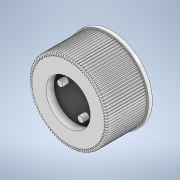
# Autodesk Inventor part: 100ml Bottle 2 lid
Saved by Autodesk Inventor 2021 (Build 250183000, 183)
## iProperties
Created: 2019-11-05
Part Number: 100ml Bottle 2 lid
Material: Generic
Document SubType Name: Modeling
Designer: jgray
Density: 1 g/cm^3
Appearance: Default
Author: jgray
Autodesk Inventor part; units mm, degrees
ref_plane "YZ Plane" through (0, 0, 0) normal (1, 0, 0) x (0, 1, 0)
ref_plane "XZ Plane" through (0, 0, 0) normal (0, 1, 0) x (-1, 0, 0)
ref_plane "XY Plane" through (0, 0, 0) normal (0, 0, 1) x (1, 0, 0)
sketch "Sketch1" plane through (0, 0, 0) normal (0, 0, 1) x (1, 0, 0)
  circle A0 centre (0, 0) radius 13.8
  dimension "d0" = 27.6
  constraints: 1 centre point, 1 coincident
  measures "d0" diameter of A0
extrude "Extrusion1" add sketch "Sketch1" along normal blind 1.3
sketch "Sketch2" plane through (0, 0, 1.3) normal (0, 0, 1) x (1, 0, 0)
  circle A0 centre (0, 0) radius 13.4
  circle A1 centre (0, 0) radius 12.9 construction
  line L0 (0, 13.4) -> (0.8414, 13.3736) construction
  line L1 (0.8414, 13.3736) -> (1.6795, 13.2943) construction
  line L2 (1.6795, 13.2943) -> (2.5109, 13.1626) construction
  line L3 (2.5109, 13.1626) -> (3.3324, 12.979) construction
  line L4 (3.3324, 12.979) -> (4.1408, 12.7442) construction
  line L5 (4.1408, 12.7442) -> (4.9329, 12.459) construction
  line L6 (4.9329, 12.459) -> (5.7054, 12.1247) construction
  line L7 (5.7054, 12.1247) -> (6.4555, 11.7425) construction
  line L8 (6.4555, 11.7425) -> (7.1801, 11.314) construction
  line L9 (7.1801, 11.314) -> (7.8763, 10.8408) construction
  line L10 (7.8763, 10.8408) -> (8.5415, 10.3249) construction
  line L11 (8.5415, 10.3249) -> (9.1729, 9.7682) construction
  line L12 (9.1729, 9.7682) -> (9.7682, 9.1729) construction
  line L13 (9.7682, 9.1729) -> (10.3249, 8.5415) construction
  line L14 (10.3249, 8.5415) -> (10.8408, 7.8763) construction
  line L15 (10.8408, 7.8763) -> (11.314, 7.1801) construction
  line L16 (11.314, 7.1801) -> (11.7425, 6.4555) construction
  line L17 (11.7425, 6.4555) -> (12.1247, 5.7054) construction
  line L18 (12.1247, 5.7054) -> (12.459, 4.9329) construction
  line L19 (12.459, 4.9329) -> (12.7442, 4.1408) construction
  line L20 (12.7442, 4.1408) -> (12.979, 3.3324) construction
  line L21 (12.979, 3.3324) -> (13.1626, 2.5109) construction
  line L22 (13.1626, 2.5109) -> (13.2943, 1.6795) construction
  line L23 (13.2943, 1.6795) -> (13.3736, 0.8414) construction
  line L24 (13.3736, 0.8414) -> (13.4, 0) construction
  line L25 (13.4, 0) -> (13.3736, -0.8414) construction
  line L26 (13.3736, -0.8414) -> (13.2943, -1.6795) construction
  line L27 (13.2943, -1.6795) -> (13.1626, -2.5109) construction
  line L28 (13.1626, -2.5109) -> (12.979, -3.3324) construction
  line L29 (12.979, -3.3324) -> (12.7442, -4.1408) construction
  line L30 (12.7442, -4.1408) -> (12.459, -4.9329) construction
  line L31 (12.459, -4.9329) -> (12.1247, -5.7054) construction
  line L32 (12.1247, -5.7054) -> (11.7425, -6.4555) construction
  line L33 (11.7425, -6.4555) -> (11.314, -7.1801) construction
  line L34 (11.314, -7.1801) -> (10.8408, -7.8763) construction
  line L35 (10.8408, -7.8763) -> (10.3249, -8.5415) construction
  line L36 (10.3249, -8.5415) -> (9.7682, -9.1729) construction
  line L37 (9.7682, -9.1729) -> (9.1729, -9.7682) construction
  line L38 (9.1729, -9.7682) -> (8.5415, -10.3249) construction
  line L39 (8.5415, -10.3249) -> (7.8763, -10.8408) construction
  line L40 (7.8763, -10.8408) -> (7.1801, -11.314) construction
  line L41 (7.1801, -11.314) -> (6.4555, -11.7425) construction
  line L42 (6.4555, -11.7425) -> (5.7054, -12.1247) construction
  line L43 (5.7054, -12.1247) -> (4.9329, -12.459) construction
  line L44 (4.9329, -12.459) -> (4.1408, -12.7442) construction
  line L45 (4.1408, -12.7442) -> (3.3324, -12.979) construction
  line L46 (3.3324, -12.979) -> (2.5109, -13.1626) construction
  line L47 (2.5109, -13.1626) -> (1.6795, -13.2943) construction
  line L48 (1.6795, -13.2943) -> (0.8414, -13.3736) construction
  line L49 (0.8414, -13.3736) -> (0, -13.4) construction
  line L50 (0, -13.4) -> (-0.8414, -13.3736) construction
  line L51 (-0.8414, -13.3736) -> (-1.6795, -13.2943) construction
  line L52 (-1.6795, -13.2943) -> (-2.5109, -13.1626) construction
  line L53 (-2.5109, -13.1626) -> (-3.3324, -12.979) construction
  line L54 (-3.3324, -12.979) -> (-4.1408, -12.7442) construction
  line L55 (-4.1408, -12.7442) -> (-4.9329, -12.459) construction
  line L56 (-4.9329, -12.459) -> (-5.7054, -12.1247) construction
  line L57 (-5.7054, -12.1247) -> (-6.4555, -11.7425) construction
  line L58 (-6.4555, -11.7425) -> (-7.1801, -11.314) construction
  line L59 (-7.1801, -11.314) -> (-7.8763, -10.8408) construction
  line L60 (-7.8763, -10.8408) -> (-8.5415, -10.3249) construction
  line L61 (-8.5415, -10.3249) -> (-9.1729, -9.7682) construction
  line L62 (-9.1729, -9.7682) -> (-9.7682, -9.1729) construction
  line L63 (-9.7682, -9.1729) -> (-10.3249, -8.5415) construction
  line L64 (-10.3249, -8.5415) -> (-10.8408, -7.8763) construction
  line L65 (-10.8408, -7.8763) -> (-11.314, -7.1801) construction
  line L66 (-11.314, -7.1801) -> (-11.7425, -6.4555) construction
  line L67 (-11.7425, -6.4555) -> (-12.1247, -5.7054) construction
  line L68 (-12.1247, -5.7054) -> (-12.459, -4.9329) construction
  line L69 (-12.459, -4.9329) -> (-12.7442, -4.1408) construction
  line L70 (-12.7442, -4.1408) -> (-12.979, -3.3324) construction
  line L71 (-12.979, -3.3324) -> (-13.1626, -2.5109) construction
  line L72 (-13.1626, -2.5109) -> (-13.2943, -1.6795) construction
  line L73 (-13.2943, -1.6795) -> (-13.3736, -0.8414) construction
  line L74 (-13.3736, -0.8414) -> (-13.4, 0) construction
  line L75 (-13.4, 0) -> (-13.3736, 0.8414) construction
  line L76 (-13.3736, 0.8414) -> (-13.2943, 1.6795) construction
  line L77 (-13.2943, 1.6795) -> (-13.1626, 2.5109) construction
  line L78 (-13.1626, 2.5109) -> (-12.979, 3.3324) construction
  line L79 (-12.979, 3.3324) -> (-12.7442, 4.1408) construction
  line L80 (-12.7442, 4.1408) -> (-12.459, 4.9329) construction
  line L81 (-12.459, 4.9329) -> (-12.1247, 5.7054) construction
  line L82 (-12.1247, 5.7054) -> (-11.7425, 6.4555) construction
  line L83 (-11.7425, 6.4555) -> (-11.314, 7.1801) construction
  line L84 (-11.314, 7.1801) -> (-10.8408, 7.8763) construction
  line L85 (-10.8408, 7.8763) -> (-10.3249, 8.5415) construction
  line L86 (-10.3249, 8.5415) -> (-9.7682, 9.1729) construction
  line L87 (-9.7682, 9.1729) -> (-9.1729, 9.7682) construction
  line L88 (-9.1729, 9.7682) -> (-8.5415, 10.3249) construction
  line L89 (-8.5415, 10.3249) -> (-7.8763, 10.8408) construction
  line L90 (-7.8763, 10.8408) -> (-7.1801, 11.314) construction
  line L91 (-7.1801, 11.314) -> (-6.4555, 11.7425) construction
  line L92 (-6.4555, 11.7425) -> (-5.7054, 12.1247) construction
  line L93 (-5.7054, 12.1247) -> (-4.9329, 12.459) construction
  line L94 (-4.9329, 12.459) -> (-4.1408, 12.7442) construction
  line L95 (-4.1408, 12.7442) -> (-3.3324, 12.979) construction
  line L96 (-3.3324, 12.979) -> (-2.5109, 13.1626) construction
  line L97 (-2.5109, 13.1626) -> (-1.6795, 13.2943) construction
  line L98 (-1.6795, 13.2943) -> (-0.8414, 13.3736) construction
  line L99 (-0.8414, 13.3736) -> (0, 13.4) construction
  line L100 (0, 0) -> (-0.4207, 13.3868) construction
  line L101 (-0.4052, 12.8936) -> (0.4052, 12.8936) construction
  line L102 (0.4052, 12.8936) -> (1.214, 12.8427) construction
  line L103 (1.214, 12.8427) -> (2.018, 12.7412) construction
  line L104 (2.018, 12.7412) -> (2.814, 12.5893) construction
  line L105 (2.814, 12.5893) -> (3.599, 12.3878) construction
  line L106 (3.599, 12.3878) -> (4.3697, 12.1374) construction
  line L107 (4.3697, 12.1374) -> (5.1232, 11.839) construction
  line L108 (5.1232, 11.839) -> (5.8565, 11.494) construction
  line L109 (5.8565, 11.494) -> (6.5666, 11.1036) construction
  line L110 (6.5666, 11.1036) -> (7.2509, 10.6693) construction
  line L111 (7.2509, 10.6693) -> (7.9065, 10.193) construction
  line L112 (7.9065, 10.193) -> (8.5309, 9.6764) construction
  line L113 (8.5309, 9.6764) -> (9.1217, 9.1217) construction
  line L114 (9.1217, 9.1217) -> (9.6764, 8.5309) construction
  line L115 (9.6764, 8.5309) -> (10.193, 7.9065) construction
  line L116 (10.193, 7.9065) -> (10.6693, 7.2509) construction
  line L117 (10.6693, 7.2509) -> (11.1036, 6.5666) construction
  line L118 (11.1036, 6.5666) -> (11.494, 5.8565) construction
  line L119 (11.494, 5.8565) -> (11.839, 5.1232) construction
  line L120 (11.839, 5.1232) -> (12.1374, 4.3697) construction
  line L121 (12.1374, 4.3697) -> (12.3878, 3.599) construction
  line L122 (12.3878, 3.599) -> (12.5893, 2.814) construction
  line L123 (12.5893, 2.814) -> (12.7412, 2.018) construction
  line L124 (12.7412, 2.018) -> (12.8427, 1.214) construction
  line L125 (12.8427, 1.214) -> (12.8936, 0.4052) construction
  line L126 (12.8936, 0.4052) -> (12.8936, -0.4052) construction
  line L127 (12.8936, -0.4052) -> (12.8427, -1.214) construction
  line L128 (12.8427, -1.214) -> (12.7412, -2.018) construction
  line L129 (12.7412, -2.018) -> (12.5893, -2.814) construction
  line L130 (12.5893, -2.814) -> (12.3878, -3.599) construction
  line L131 (12.3878, -3.599) -> (12.1374, -4.3697) construction
  line L132 (12.1374, -4.3697) -> (11.839, -5.1232) construction
  line L133 (11.839, -5.1232) -> (11.494, -5.8565) construction
  line L134 (11.494, -5.8565) -> (11.1036, -6.5666) construction
  line L135 (11.1036, -6.5666) -> (10.6693, -7.2509) construction
  line L136 (10.6693, -7.2509) -> (10.193, -7.9065) construction
  line L137 (10.193, -7.9065) -> (9.6764, -8.5309) construction
  line L138 (9.6764, -8.5309) -> (9.1217, -9.1217) construction
  line L139 (9.1217, -9.1217) -> (8.5309, -9.6764) construction
  line L140 (8.5309, -9.6764) -> (7.9065, -10.193) construction
  line L141 (7.9065, -10.193) -> (7.2509, -10.6693) construction
  line L142 (7.2509, -10.6693) -> (6.5666, -11.1036) construction
  line L143 (6.5666, -11.1036) -> (5.8565, -11.494) construction
  line L144 (5.8565, -11.494) -> (5.1232, -11.839) construction
  line L145 (5.1232, -11.839) -> (4.3697, -12.1374) construction
  line L146 (4.3697, -12.1374) -> (3.599, -12.3878) construction
  line L147 (3.599, -12.3878) -> (2.814, -12.5893) construction
  line L148 (2.814, -12.5893) -> (2.018, -12.7412) construction
  line L149 (2.018, -12.7412) -> (1.214, -12.8427) construction
  line L150 (1.214, -12.8427) -> (0.4052, -12.8936) construction
  line L151 (0.4052, -12.8936) -> (-0.4052, -12.8936) construction
  line L152 (-0.4052, -12.8936) -> (-1.214, -12.8427) construction
  line L153 (-1.214, -12.8427) -> (-2.018, -12.7412) construction
  line L154 (-2.018, -12.7412) -> (-2.814, -12.5893) construction
  line L155 (-2.814, -12.5893) -> (-3.599, -12.3878) construction
  line L156 (-3.599, -12.3878) -> (-4.3697, -12.1374) construction
  line L157 (-4.3697, -12.1374) -> (-5.1232, -11.839) construction
  line L158 (-5.1232, -11.839) -> (-5.8565, -11.494) construction
  line L159 (-5.8565, -11.494) -> (-6.5666, -11.1036) construction
  line L160 (-6.5666, -11.1036) -> (-7.2509, -10.6693) construction
  line L161 (-7.2509, -10.6693) -> (-7.9065, -10.193) construction
  line L162 (-7.9065, -10.193) -> (-8.5309, -9.6764) construction
  line L163 (-8.5309, -9.6764) -> (-9.1217, -9.1217) construction
  line L164 (-9.1217, -9.1217) -> (-9.6764, -8.5309) construction
  line L165 (-9.6764, -8.5309) -> (-10.193, -7.9065) construction
  line L166 (-10.193, -7.9065) -> (-10.6693, -7.2509) construction
  line L167 (-10.6693, -7.2509) -> (-11.1036, -6.5666) construction
  line L168 (-11.1036, -6.5666) -> (-11.494, -5.8565) construction
  line L169 (-11.494, -5.8565) -> (-11.839, -5.1232) construction
  line L170 (-11.839, -5.1232) -> (-12.1374, -4.3697) construction
  line L171 (-12.1374, -4.3697) -> (-12.3878, -3.599) construction
  line L172 (-12.3878, -3.599) -> (-12.5893, -2.814) construction
  line L173 (-12.5893, -2.814) -> (-12.7412, -2.018) construction
  line L174 (-12.7412, -2.018) -> (-12.8427, -1.214) construction
  line L175 (-12.8427, -1.214) -> (-12.8936, -0.4052) construction
  line L176 (-12.8936, -0.4052) -> (-12.8936, 0.4052) construction
  line L177 (-12.8936, 0.4052) -> (-12.8427, 1.214) construction
  line L178 (-12.8427, 1.214) -> (-12.7412, 2.018) construction
  line L179 (-12.7412, 2.018) -> (-12.5893, 2.814) construction
  line L180 (-12.5893, 2.814) -> (-12.3878, 3.599) construction
  line L181 (-12.3878, 3.599) -> (-12.1374, 4.3697) construction
  line L182 (-12.1374, 4.3697) -> (-11.839, 5.1232) construction
  line L183 (-11.839, 5.1232) -> (-11.494, 5.8565) construction
  line L184 (-11.494, 5.8565) -> (-11.1036, 6.5666) construction
  line L185 (-11.1036, 6.5666) -> (-10.6693, 7.2509) construction
  line L186 (-10.6693, 7.2509) -> (-10.193, 7.9065) construction
  line L187 (-10.193, 7.9065) -> (-9.6764, 8.5309) construction
  line L188 (-9.6764, 8.5309) -> (-9.1217, 9.1217) construction
  line L189 (-9.1217, 9.1217) -> (-8.5309, 9.6764) construction
  line L190 (-8.5309, 9.6764) -> (-7.9065, 10.193) construction
  line L191 (-7.9065, 10.193) -> (-7.2509, 10.6693) construction
  line L192 (-7.2509, 10.6693) -> (-6.5666, 11.1036) construction
  line L193 (-6.5666, 11.1036) -> (-5.8565, 11.494) construction
  line L194 (-5.8565, 11.494) -> (-5.1232, 11.839) construction
  line L195 (-5.1232, 11.839) -> (-4.3697, 12.1374) construction
  line L196 (-4.3697, 12.1374) -> (-3.599, 12.3878) construction
  line L197 (-3.599, 12.3878) -> (-2.814, 12.5893) construction
  line L198 (-2.814, 12.5893) -> (-2.018, 12.7412) construction
  line L199 (-2.018, 12.7412) -> (-1.214, 12.8427) construction
  line L200 (-1.214, 12.8427) -> (-0.4052, 12.8936) construction
  line L201 (-0.4052, 12.8936) -> (0, 13.3868)
  line L202 (0, 13.3868) -> (0.4052, 12.8936)
  line L203 (-1.214, 12.8427) -> (-0.8406, 13.3604)
  line L204 (-0.8406, 13.3604) -> (-0.4052, 12.8936)
  line L205 (-2.018, 12.7412) -> (-1.6778, 13.2812)
  line L206 (-1.6778, 13.2812) -> (-1.214, 12.8427)
  line L207 (-2.814, 12.5893) -> (-2.5084, 13.1497)
  line L208 (-2.5084, 13.1497) -> (-2.018, 12.7412)
  line L209 (-3.599, 12.3878) -> (-3.3292, 12.9662)
  line L210 (-3.3292, 12.9662) -> (-2.814, 12.5893)
  line L211 (-4.3697, 12.1374) -> (-4.1367, 12.7316)
  line L212 (-4.1367, 12.7316) -> (-3.599, 12.3878)
  line L213 (-5.1232, 11.839) -> (-4.928, 12.4467)
  line L214 (-4.928, 12.4467) -> (-4.3697, 12.1374)
  line L215 (-5.8565, 11.494) -> (-5.6998, 12.1127)
  line L216 (-5.6998, 12.1127) -> (-5.1232, 11.839)
  line L217 (-6.5666, 11.1036) -> (-6.4491, 11.7309)
  line L218 (-6.4491, 11.7309) -> (-5.8565, 11.494)
  line L219 (-7.2509, 10.6693) -> (-7.173, 11.3028)
  line L220 (-7.173, 11.3028) -> (-6.5666, 11.1036)
  line L221 (-7.9065, 10.193) -> (-7.8686, 10.8301)
  line L222 (-7.8686, 10.8301) -> (-7.2509, 10.6693)
  line L223 (-8.5309, 9.6764) -> (-8.5331, 10.3147)
  line L224 (-8.5331, 10.3147) -> (-7.9065, 10.193)
  line L225 (-9.1217, 9.1217) -> (-9.1639, 9.7585)
  line L226 (-9.1639, 9.7585) -> (-8.5309, 9.6764)
  line L227 (-9.6764, 8.5309) -> (-9.7585, 9.1639)
  line L228 (-9.7585, 9.1639) -> (-9.1217, 9.1217)
  line L229 (-10.193, 7.9065) -> (-10.3147, 8.5331)
  line L230 (-10.3147, 8.5331) -> (-9.6764, 8.5309)
  line L231 (-10.6693, 7.2509) -> (-10.8301, 7.8686)
  line L232 (-10.8301, 7.8686) -> (-10.193, 7.9065)
  line L233 (-11.1036, 6.5666) -> (-11.3028, 7.173)
  line L234 (-11.3028, 7.173) -> (-10.6693, 7.2509)
  line L235 (-11.494, 5.8565) -> (-11.7309, 6.4491)
  line L236 (-11.7309, 6.4491) -> (-11.1036, 6.5666)
  line L237 (-11.839, 5.1232) -> (-12.1127, 5.6998)
  line L238 (-12.1127, 5.6998) -> (-11.494, 5.8565)
  line L239 (-12.1374, 4.3697) -> (-12.4467, 4.928)
  line L240 (-12.4467, 4.928) -> (-11.839, 5.1232)
  line L241 (-12.3878, 3.599) -> (-12.7316, 4.1367)
  line L242 (-12.7316, 4.1367) -> (-12.1374, 4.3697)
  line L243 (-12.5893, 2.814) -> (-12.9662, 3.3292)
  line L244 (-12.9662, 3.3292) -> (-12.3878, 3.599)
  line L245 (-12.7412, 2.018) -> (-13.1497, 2.5084)
  line L246 (-13.1497, 2.5084) -> (-12.5893, 2.814)
  line L247 (-12.8427, 1.214) -> (-13.2812, 1.6778)
  line L248 (-13.2812, 1.6778) -> (-12.7412, 2.018)
  line L249 (-12.8936, 0.4052) -> (-13.3604, 0.8406)
  line L250 (-13.3604, 0.8406) -> (-12.8427, 1.214)
  line L251 (-12.8936, -0.4052) -> (-13.3868, 0)
  line L252 (-13.3868, 0) -> (-12.8936, 0.4052)
  line L253 (-12.8427, -1.214) -> (-13.3604, -0.8406)
  line L254 (-13.3604, -0.8406) -> (-12.8936, -0.4052)
  line L255 (-12.7412, -2.018) -> (-13.2812, -1.6778)
  line L256 (-13.2812, -1.6778) -> (-12.8427, -1.214)
  line L257 (-12.5893, -2.814) -> (-13.1497, -2.5084)
  line L258 (-13.1497, -2.5084) -> (-12.7412, -2.018)
  line L259 (-12.3878, -3.599) -> (-12.9662, -3.3292)
  line L260 (-12.9662, -3.3292) -> (-12.5893, -2.814)
  line L261 (-12.1374, -4.3697) -> (-12.7316, -4.1367)
  line L262 (-12.7316, -4.1367) -> (-12.3878, -3.599)
  line L263 (-11.839, -5.1232) -> (-12.4467, -4.928)
  line L264 (-12.4467, -4.928) -> (-12.1374, -4.3697)
  line L265 (-11.494, -5.8565) -> (-12.1127, -5.6998)
  line L266 (-12.1127, -5.6998) -> (-11.839, -5.1232)
  line L267 (-11.1036, -6.5666) -> (-11.7309, -6.4491)
  line L268 (-11.7309, -6.4491) -> (-11.494, -5.8565)
  line L269 (-10.6693, -7.2509) -> (-11.3028, -7.173)
  line L270 (-11.3028, -7.173) -> (-11.1036, -6.5666)
  line L271 (-10.193, -7.9065) -> (-10.8301, -7.8686)
  line L272 (-10.8301, -7.8686) -> (-10.6693, -7.2509)
  line L273 (-9.6764, -8.5309) -> (-10.3147, -8.5331)
  line L274 (-10.3147, -8.5331) -> (-10.193, -7.9065)
  line L275 (-9.1217, -9.1217) -> (-9.7585, -9.1639)
  line L276 (-9.7585, -9.1639) -> (-9.6764, -8.5309)
  line L277 (-8.5309, -9.6764) -> (-9.1639, -9.7585)
  line L278 (-9.1639, -9.7585) -> (-9.1217, -9.1217)
  line L279 (-7.9065, -10.193) -> (-8.5331, -10.3147)
  line L280 (-8.5331, -10.3147) -> (-8.5309, -9.6764)
  line L281 (-7.2509, -10.6693) -> (-7.8686, -10.8301)
  line L282 (-7.8686, -10.8301) -> (-7.9065, -10.193)
  line L283 (-6.5666, -11.1036) -> (-7.173, -11.3028)
  line L284 (-7.173, -11.3028) -> (-7.2509, -10.6693)
  line L285 (-5.8565, -11.494) -> (-6.4491, -11.7309)
  line L286 (-6.4491, -11.7309) -> (-6.5666, -11.1036)
  line L287 (-5.1232, -11.839) -> (-5.6998, -12.1127)
  line L288 (-5.6998, -12.1127) -> (-5.8565, -11.494)
  line L289 (-4.3697, -12.1374) -> (-4.928, -12.4467)
  line L290 (-4.928, -12.4467) -> (-5.1232, -11.839)
  line L291 (-3.599, -12.3878) -> (-4.1367, -12.7316)
  line L292 (-4.1367, -12.7316) -> (-4.3697, -12.1374)
  line L293 (-2.814, -12.5893) -> (-3.3292, -12.9662)
  line L294 (-3.3292, -12.9662) -> (-3.599, -12.3878)
  line L295 (-2.018, -12.7412) -> (-2.5084, -13.1497)
  line L296 (-2.5084, -13.1497) -> (-2.814, -12.5893)
  line L297 (-1.214, -12.8427) -> (-1.6778, -13.2812)
  line L298 (-1.6778, -13.2812) -> (-2.018, -12.7412)
  line L299 (-0.4052, -12.8936) -> (-0.8406, -13.3604)
  line L300 (-0.8406, -13.3604) -> (-1.214, -12.8427)
  line L301 (0.4052, -12.8936) -> (0, -13.3868)
  line L302 (0, -13.3868) -> (-0.4052, -12.8936)
  line L303 (1.214, -12.8427) -> (0.8406, -13.3604)
  line L304 (0.8406, -13.3604) -> (0.4052, -12.8936)
  line L305 (2.018, -12.7412) -> (1.6778, -13.2812)
  line L306 (1.6778, -13.2812) -> (1.214, -12.8427)
  line L307 (2.814, -12.5893) -> (2.5084, -13.1497)
  line L308 (2.5084, -13.1497) -> (2.018, -12.7412)
  line L309 (3.599, -12.3878) -> (3.3292, -12.9662)
  line L310 (3.3292, -12.9662) -> (2.814, -12.5893)
  line L311 (4.3697, -12.1374) -> (4.1367, -12.7316)
  line L312 (4.1367, -12.7316) -> (3.599, -12.3878)
  line L313 (5.1232, -11.839) -> (4.928, -12.4467)
  line L314 (4.928, -12.4467) -> (4.3697, -12.1374)
  line L315 (5.8565, -11.494) -> (5.6998, -12.1127)
  line L316 (5.6998, -12.1127) -> (5.1232, -11.839)
  line L317 (6.5666, -11.1036) -> (6.4491, -11.7309)
  line L318 (6.4491, -11.7309) -> (5.8565, -11.494)
  line L319 (7.2509, -10.6693) -> (7.173, -11.3028)
  line L320 (7.173, -11.3028) -> (6.5666, -11.1036)
  line L321 (7.9065, -10.193) -> (7.8686, -10.8301)
  line L322 (7.8686, -10.8301) -> (7.2509, -10.6693)
  line L323 (8.5309, -9.6764) -> (8.5331, -10.3147)
  line L324 (8.5331, -10.3147) -> (7.9065, -10.193)
  line L325 (9.1217, -9.1217) -> (9.1639, -9.7585)
  line L326 (9.1639, -9.7585) -> (8.5309, -9.6764)
  line L327 (9.6764, -8.5309) -> (9.7585, -9.1639)
  line L328 (9.7585, -9.1639) -> (9.1217, -9.1217)
  line L329 (10.193, -7.9065) -> (10.3147, -8.5331)
  line L330 (10.3147, -8.5331) -> (9.6764, -8.5309)
  line L331 (10.6693, -7.2509) -> (10.8301, -7.8686)
  line L332 (10.8301, -7.8686) -> (10.193, -7.9065)
  line L333 (11.1036, -6.5666) -> (11.3028, -7.173)
  line L334 (11.3028, -7.173) -> (10.6693, -7.2509)
  line L335 (11.494, -5.8565) -> (11.7309, -6.4491)
  line L336 (11.7309, -6.4491) -> (11.1036, -6.5666)
  line L337 (11.839, -5.1232) -> (12.1127, -5.6998)
  line L338 (12.1127, -5.6998) -> (11.494, -5.8565)
  line L339 (12.1374, -4.3697) -> (12.4467, -4.928)
  line L340 (12.4467, -4.928) -> (11.839, -5.1232)
  line L341 (12.3878, -3.599) -> (12.7316, -4.1367)
  line L342 (12.7316, -4.1367) -> (12.1374, -4.3697)
  line L343 (12.5893, -2.814) -> (12.9662, -3.3292)
  line L344 (12.9662, -3.3292) -> (12.3878, -3.599)
  line L345 (12.7412, -2.018) -> (13.1497, -2.5084)
  line L346 (13.1497, -2.5084) -> (12.5893, -2.814)
  line L347 (12.8427, -1.214) -> (13.2812, -1.6778)
  line L348 (13.2812, -1.6778) -> (12.7412, -2.018)
  line L349 (12.8936, -0.4052) -> (13.3604, -0.8406)
  line L350 (13.3604, -0.8406) -> (12.8427, -1.214)
  line L351 (12.8936, 0.4052) -> (13.3868, 0)
  line L352 (13.3868, 0) -> (12.8936, -0.4052)
  line L353 (12.8427, 1.214) -> (13.3604, 0.8406)
  line L354 (13.3604, 0.8406) -> (12.8936, 0.4052)
  line L355 (12.7412, 2.018) -> (13.2812, 1.6778)
  line L356 (13.2812, 1.6778) -> (12.8427, 1.214)
  line L357 (12.5893, 2.814) -> (13.1497, 2.5084)
  line L358 (13.1497, 2.5084) -> (12.7412, 2.018)
  line L359 (12.3878, 3.599) -> (12.9662, 3.3292)
  line L360 (12.9662, 3.3292) -> (12.5893, 2.814)
  line L361 (12.1374, 4.3697) -> (12.7316, 4.1367)
  line L362 (12.7316, 4.1367) -> (12.3878, 3.599)
  line L363 (11.839, 5.1232) -> (12.4467, 4.928)
  line L364 (12.4467, 4.928) -> (12.1374, 4.3697)
  line L365 (11.494, 5.8565) -> (12.1127, 5.6998)
  line L366 (12.1127, 5.6998) -> (11.839, 5.1232)
  line L367 (11.1036, 6.5666) -> (11.7309, 6.4491)
  line L368 (11.7309, 6.4491) -> (11.494, 5.8565)
  line L369 (10.6693, 7.2509) -> (11.3028, 7.173)
  line L370 (11.3028, 7.173) -> (11.1036, 6.5666)
  line L371 (10.193, 7.9065) -> (10.8301, 7.8686)
  line L372 (10.8301, 7.8686) -> (10.6693, 7.2509)
  line L373 (9.6764, 8.5309) -> (10.3147, 8.5331)
  line L374 (10.3147, 8.5331) -> (10.193, 7.9065)
  line L375 (9.1217, 9.1217) -> (9.7585, 9.1639)
  line L376 (9.7585, 9.1639) -> (9.6764, 8.5309)
  line L377 (8.5309, 9.6764) -> (9.1639, 9.7585)
  line L378 (9.1639, 9.7585) -> (9.1217, 9.1217)
  line L379 (7.9065, 10.193) -> (8.5331, 10.3147)
  line L380 (8.5331, 10.3147) -> (8.5309, 9.6764)
  line L381 (7.2509, 10.6693) -> (7.8686, 10.8301)
  line L382 (7.8686, 10.8301) -> (7.9065, 10.193)
  line L383 (6.5666, 11.1036) -> (7.173, 11.3028)
  line L384 (7.173, 11.3028) -> (7.2509, 10.6693)
  line L385 (5.8565, 11.494) -> (6.4491, 11.7309)
  line L386 (6.4491, 11.7309) -> (6.5666, 11.1036)
  line L387 (5.1232, 11.839) -> (5.6998, 12.1127)
  line L388 (5.6998, 12.1127) -> (5.8565, 11.494)
  line L389 (4.3697, 12.1374) -> (4.928, 12.4467)
  line L390 (4.928, 12.4467) -> (5.1232, 11.839)
  line L391 (3.599, 12.3878) -> (4.1367, 12.7316)
  line L392 (4.1367, 12.7316) -> (4.3697, 12.1374)
  line L393 (2.814, 12.5893) -> (3.3292, 12.9662)
  line L394 (3.3292, 12.9662) -> (3.599, 12.3878)
  line L395 (2.018, 12.7412) -> (2.5084, 13.1497)
  line L396 (2.5084, 13.1497) -> (2.814, 12.5893)
  line L397 (1.214, 12.8427) -> (1.6778, 13.2812)
  line L398 (1.6778, 13.2812) -> (2.018, 12.7412)
  line L399 (0.4052, 12.8936) -> (0.8406, 13.3604)
  line L400 (0.8406, 13.3604) -> (1.214, 12.8427)
  dimension "d3" = 26.8
  dimension "d4" = 25.8
  dimension "d7" = 360
  constraints: 802 end point, 4 coincident, 2 point on circle, 2 point on line, 1 centre point, 1 midpoint, 1 vertical alignment, 905 other
  measures "d4" diameter of A1
extrude "Extrusion2" add sketch "Sketch2" along normal blind 13.5 contours L201 L202 L399 L400 L397 L398 L395 L396 L393 L394 L391 L392 L389 L390 L387 L388 L385 L386 L383 L384 L381 L382 L379 L380 L377 L378 L375 L376 L373 L374 L371 L372 L369 L370 L367 L368 L365 L366 L363 L364 L361 L362 L359 L360 L357 L358 L355 L356 L353 L354 L351 L352 L349 L350 L347 L348 L345 L346 L343 L344 L341 L342 L339 L340 L337 L338 L335 L336 L333 L334 L331 L332 L329 L330 L327 L328 L325 L326 L323 L324 L321 L322 L319 L320 L317 L318 L315 L316 L313 L314 L311 L312 L309 L310 L307 L308 L305 L306 L303 L304 L301 L302 L299 L300 L297 L298 L295 L296 L293 L294 L291 L292 L289 L290 L287 L288 L285 L286 L283 L284 L281 L282 L279 L280 L277 L278 L275 L276 L273 L274 L271 L272 L269 L270 L267 L268 L265 L266 L263 L264 L261 L262 L259 L260 L257 L258 L255 L256 L253 L254 L251 L252 L249 L250 L247 L248 L245 L246 L243 L244 L241 L242 L239 L240 L237 L238 L235 L236 L233 L234 L231 L232 L229 L230 L227 L228 L225 L226 L223 L224 L221 L222 L219 L220 L217 L218 L215 L216 L213 L214 L211 L212 L209 L210 L207 L208 L205 L206 L203 L204
sketch "Sketch3" plane through (0, 0, 14.8) normal (0, 0, 1) x (1, 0, 0)
  circle A0 centre (0, 0) radius 13.3868
  constraints: 1 centre point, 1 coincident
fillet "Fillet1" radius 0.5 200 edges at (10.5116, -7.8875, 14.8) (10.7497, -7.5597, 14.8) (10.9861, -7.2119, 14.8) (11.2032, -6.8698, 14.8) (11.4172, -6.5079, 14.8) (11.6125, -6.1528, 14.8) (11.8034, -5.7781, 14.8) (11.9759, -5.4115, 14.8) (12.1429, -5.0256, 14.8) (12.292, -4.6489, 14.8) (12.4345, -4.2532, 14.8) (12.5597, -3.8679, 14.8) (12.677, -3.4641, 14.8) (12.7778, -3.0716, 14.8) (12.8695, -2.6612, 14.8) (12.9454, -2.2632, 14.8) (13.0112, -1.8479, 14.8) (13.062, -1.4459, 14.8) (13.1016, -1.0273, 14.8) (13.127, -0.6229, 14.8) (13.1402, -0.2026, 14.8) (13.1402, 0.2026, 14.8) (13.127, 0.6229, 14.8) (13.1016, 1.0273, 14.8) (13.062, 1.4459, 14.8) (13.0112, 1.8479, 14.8) (12.9454, 2.2632, 14.8) (12.8695, 2.6612, 14.8) (12.7778, 3.0716, 14.8) (12.677, 3.4641, 14.8) (12.5597, 3.8679, 14.8) (12.4345, 4.2532, 14.8) (12.292, 4.6489, 14.8) (12.1429, 5.0256, 14.8) (11.9759, 5.4115, 14.8) (11.8034, 5.7781, 14.8) (11.6125, 6.1528, 14.8) (11.4172, 6.5079, 14.8) (11.2032, 6.8698, 14.8) (10.9861, 7.2119, 14.8) (10.7497, 7.5597, 14.8) (10.5116, 7.8875, 14.8) (10.2538, 8.2198, 14.8) (9.9956, 8.532, 14.8) (9.7175, 8.8474, 14.8) (9.4401, 9.1428, 14.8) (9.1428, 9.4401, 14.8) (8.8474, 9.7175, 14.8) (8.532, 9.9956, 14.8) (8.2198, 10.2538, 14.8) (7.8875, 10.5116, 14.8) (7.5597, 10.7497, 14.8) (7.2119, 10.9861, 14.8) (6.8698, 11.2032, 14.8) (6.5079, 11.4172, 14.8) (6.1528, 11.6125, 14.8) (5.7781, 11.8034, 14.8) (5.4115, 11.9759, 14.8) (5.0256, 12.1429, 14.8) (4.6489, 12.292, 14.8) (4.2532, 12.4345, 14.8) (3.8679, 12.5597, 14.8) (3.4641, 12.677, 14.8) (3.0716, 12.7778, 14.8) (2.6612, 12.8695, 14.8) (2.2632, 12.9454, 14.8) (1.8479, 13.0112, 14.8) (1.4459, 13.062, 14.8) (1.0273, 13.1016, 14.8) (0.6229, 13.127, 14.8) (0.2026, 13.1402, 14.8) (-0.2026, 13.1402, 14.8) (-0.6229, 13.127, 14.8) (-1.0273, 13.1016, 14.8) (-1.4459, 13.062, 14.8) (-1.8479, 13.0112, 14.8) (-2.2632, 12.9454, 14.8) (-2.6612, 12.8695, 14.8) (-3.0716, 12.7778, 14.8) (-3.4641, 12.677, 14.8) (-3.8679, 12.5597, 14.8) (-4.2532, 12.4345, 14.8) (-4.6489, 12.292, 14.8) (-5.0256, 12.1429, 14.8) (-5.4115, 11.9759, 14.8) (-5.7781, 11.8034, 14.8) (-6.1528, 11.6125, 14.8) (-6.5079, 11.4172, 14.8) (-6.8698, 11.2032, 14.8) (-7.2119, 10.9861, 14.8) (-7.5597, 10.7497, 14.8) (-7.8875, 10.5116, 14.8) (-8.2198, 10.2538, 14.8) (-8.532, 9.9956, 14.8) (-8.8474, 9.7175, 14.8) (-9.1428, 9.4401, 14.8) (-9.4401, 9.1428, 14.8) (-9.7175, 8.8474, 14.8) (-9.9956, 8.532, 14.8) (-10.2538, 8.2198, 14.8) (-10.5116, 7.8875, 14.8) (-10.7497, 7.5597, 14.8) (-10.9861, 7.2119, 14.8) (-11.2032, 6.8698, 14.8) (-11.4172, 6.5079, 14.8) (-11.6125, 6.1528, 14.8) (-11.8034, 5.7781, 14.8) (-11.9759, 5.4115, 14.8) (-12.1429, 5.0256, 14.8) (-12.292, 4.6489, 14.8) (-12.4345, 4.2532, 14.8) (-12.5597, 3.8679, 14.8) (-12.677, 3.4641, 14.8) (-12.7778, 3.0716, 14.8) (-12.8695, 2.6612, 14.8) (-12.9454, 2.2632, 14.8) (-13.0112, 1.8479, 14.8) (-13.062, 1.4459, 14.8) (-13.1016, 1.0273, 14.8) (-13.127, 0.6229, 14.8) (-13.1402, 0.2026, 14.8) (-13.1402, -0.2026, 14.8) (-13.127, -0.6229, 14.8) (-13.1016, -1.0273, 14.8) (-13.062, -1.4459, 14.8) (-13.0112, -1.8479, 14.8) (-12.9454, -2.2632, 14.8) (-12.8695, -2.6612, 14.8) (-12.7778, -3.0716, 14.8) (-12.677, -3.4641, 14.8) (-12.5597, -3.8679, 14.8) (-12.4345, -4.2532, 14.8) (-12.292, -4.6489, 14.8) (-12.1429, -5.0256, 14.8) (-11.9759, -5.4115, 14.8) (-11.8034, -5.7781, 14.8) (-11.6125, -6.1528, 14.8) (-11.4172, -6.5079, 14.8) (-11.2032, -6.8698, 14.8) (-10.9861, -7.2119, 14.8) (-10.7497, -7.5597, 14.8) (-10.5116, -7.8875, 14.8) (-10.2538, -8.2198, 14.8) (-9.9956, -8.532, 14.8) (-9.7175, -8.8474, 14.8) (-9.4401, -9.1428, 14.8) (-9.1428, -9.4401, 14.8) (-8.8474, -9.7175, 14.8) (-8.532, -9.9956, 14.8) (-8.2198, -10.2538, 14.8) (-7.8875, -10.5116, 14.8) (-7.5597, -10.7497, 14.8) (-7.2119, -10.9861, 14.8) (-6.8698, -11.2032, 14.8) (-6.5079, -11.4172, 14.8) (-6.1528, -11.6125, 14.8) (-5.7781, -11.8034, 14.8) (-5.4115, -11.9759, 14.8) (-5.0256, -12.1429, 14.8) (-4.6489, -12.292, 14.8) (-4.2532, -12.4345, 14.8) (-3.8679, -12.5597, 14.8) (-3.4641, -12.677, 14.8) (-3.0716, -12.7778, 14.8) (-2.6612, -12.8695, 14.8) (-2.2632, -12.9454, 14.8) (-1.8479, -13.0112, 14.8) (-1.4459, -13.062, 14.8) (-1.0273, -13.1016, 14.8) (-0.6229, -13.127, 14.8) (-0.2026, -13.1402, 14.8) (0.2026, -13.1402, 14.8) (0.6229, -13.127, 14.8) (1.0273, -13.1016, 14.8) (1.4459, -13.062, 14.8) (1.8479, -13.0112, 14.8) (2.2632, -12.9454, 14.8) (2.6612, -12.8695, 14.8) (3.0716, -12.7778, 14.8) (3.4641, -12.677, 14.8) (3.8679, -12.5597, 14.8) (4.2532, -12.4345, 14.8) (4.6489, -12.292, 14.8) (5.0256, -12.1429, 14.8) (5.4115, -11.9759, 14.8) (5.7781, -11.8034, 14.8) (6.1528, -11.6125, 14.8) (6.5079, -11.4172, 14.8) (6.8698, -11.2032, 14.8) (7.2119, -10.9861, 14.8) (7.5597, -10.7497, 14.8) (7.8875, -10.5116, 14.8) (8.2198, -10.2538, 14.8) (8.532, -9.9956, 14.8) (8.8474, -9.7175, 14.8) (9.1428, -9.4401, 14.8) (9.4401, -9.1428, 14.8) (9.7175, -8.8474, 14.8) (9.9956, -8.532, 14.8) (10.2538, -8.2198, 14.8)
sketch "Sketch4" plane through (0, 0, 14.8) normal (0, 0, 1) x (1, 0, 0)
  circle A0 centre (0, 0) radius 7.5
  dimension "d12" = 15
  constraints: 1 centre point, 1 coincident
  measures "d12" diameter of A0
extrude "Extrusion3" cut sketch "Sketch4" against normal blind 2.7
sketch "Sketch5" plane through (0, 0, 12.1) normal (0, 0, 1) x (1, 0, 0)
  line L0 (-3.5, 3.5) -> (3.5, 3.5) construction
  line L1 (3.5, 3.5) -> (3.5, -3.5) construction
  line L2 (3.5, -3.5) -> (-3.5, -3.5) construction
  line L3 (-3.5, -3.5) -> (-3.5, 3.5) construction
  circle A0 centre (-3.5, 3.5) radius 1
  circle A1 centre (3.5, -3.5) radius 1
  point P0 (0, 0)
  dimension "d15" = 7
  dimension "d16" = 7
  dimension "d17" = 3.5
  dimension "d18" = 3.5
  dimension "d19" = 2
  dimension "d20" = 2
  constraints: 8 end point, 2 centre point, 2 coincident, 2 parallel, 1 horizontal, 1 perpendicular
  measures "d15" distance of L1.end L2.end
  measures "d16" distance of L0.end L1.end
  measures "d17" distance from line of L3 point (0, 0)
  measures "d18" horizontal distance of L0.start point (0, 0)
  measures "d19" diameter of A0
  measures "d20" diameter of A1
extrude "Extrusion4" add sketch "Sketch5" along normal blind 2
body "Solid1"
